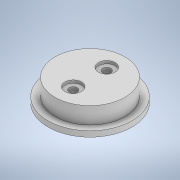
# Autodesk Inventor part: Rotor_shaft_2_2
Saved by Autodesk Inventor 2021 (Build 250183000, 183)
## iProperties
Created: 2022-08-08
Part Number: Rotor_shaft_2_2
Material: Ogólny
Document SubType Name: Modeling
Designer: MicnedSQ
Density: 1 g/cm^3
Appearance: Domyślna
Author: MicnedSQ
Autodesk Inventor part; units mm, degrees
ref_plane "YZ Plane" through (0, 0, 0) normal (1, 0, 0) x (0, 1, 0)
ref_plane "XZ Plane" through (0, 0, 0) normal (0, 1, 0) x (-1, 0, 0)
ref_plane "XY Plane" through (0, 0, 0) normal (0, 0, 1) x (1, 0, 0)
sketch "Szkic1" plane through (0, 0, 0) normal (0, 1, 0) x (-1, 0, 0)
  circle A0 centre (0, 0) radius 15
  dimension "d0" = 30
  constraints: 1 centre point, 1 coincident
  measures "d0" diameter of A0
extrude "Wyciągnięcie proste1" add sketch "Szkic1" along normal blind 2
sketch "Szkic2" plane through (0, 2, 0) normal (0, 1, 0) x (1, 0, 0)
  circle A0 centre (0, 0) radius 12.5
  dimension "d3" = 25
  constraints: 1 centre point, 1 coincident
  measures "d3" diameter of A0
extrude "Wyciągnięcie proste2" add sketch "Szkic2" along normal blind 6
sketch "Szkic3" plane through (0, 8, 0) normal (0, 1, 0) x (1, 0, 0)
  circle A0 centre (0, -6) radius 1.45
  circle A1 centre (0, 6) radius 1.45
  point P0 (0, 0)
  dimension "d6" = 2.9
  dimension "d7" = 2.9
  constraints: 2 centre point
  measures "d6" diameter of A0
  measures "d7" diameter of A1
extrude "Wyciągnięcie proste3" cut sketch "Szkic3" against normal blind 8
sketch "Szkic4" plane through (0, 0, 0) normal (0, -1, 0) x (1, 0, 0)
  arc A0 (2.12, 1.59) -> (2.12, -1.59) centre (0, 0) ccw
  line L0 (2.12, 1.59) -> (2.12, -1.59)
  dimension "d10" = 5.3
  dimension "d11" = 2.12
  constraints: 2 end point, 2 point on circle, 1 centre point, 1 coincident, 1 vertical
  measures "d10" diameter of A0
  measures "d11" distance from line of point (0, 0) L0
extrude "Wyciągnięcie proste4" cut sketch "Szkic4" against normal blind 7
sketch "Szkic5" plane through (0, 8, 0) normal (0, 1, 0) x (1, 0, 0)
  circle A0 centre (0, -6) radius 1.45 projected
  circle A1 centre (0, -6) radius 3
  circle A2 centre (0, 6) radius 1.45 projected
  circle A3 centre (0, 6) radius 3
  point P0 (0, 0)
  dimension "d14" = 6
  dimension "d15" = 6
  constraints: 2 centre point, 2 coincident
  measures "d14" diameter of A1
  measures "d15" diameter of A3
extrude "Wyciągnięcie proste5" cut sketch "Szkic5" against normal blind 1
